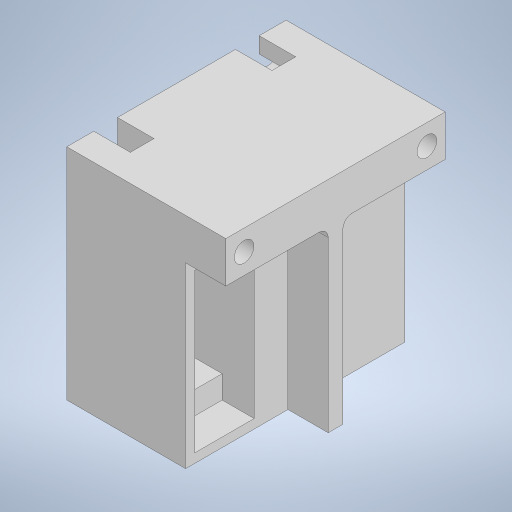
# Autodesk Inventor part: Part_2_servobox
Saved by Autodesk Inventor 2023 (Build 270158000, 158)
## iProperties
Created: 2023-09-29
Part Number: Part_2_servobox
Material: Generic
Document SubType Name: Modeling
Designer: zskus
Density: 1 g/cm^3
Appearance: Default
Author: zskus
Autodesk Inventor part; units mm, degrees
ref_plane "YZ Plane" through (0, 0, 0) normal (1, 0, 0) x (0, 1, 0)
ref_plane "XZ Plane" through (0, 0, 0) normal (0, 1, 0) x (-1, 0, 0)
ref_plane "XY Plane" through (0, 0, 0) normal (0, 0, 1) x (1, 0, 0)
sketch "Sketch1" plane through (0, 0, 0) normal (1, 0, 0) x (0, 1, 0)
  line L0 (38.1, 38.1) -> (-38.1, 38.1)
  line L1 (-38.1, 38.1) -> (-38.1, -38.1)
  line L2 (-38.1, -38.1) -> (38.1, -38.1)
  line L3 (38.1, -38.1) -> (38.1, 38.1)
  point P0 (0, 0)
  dimension "d0" = 76.2
  dimension "d1" = 76.2
  dimension "d2" = 38.1
  dimension "d3" = 38.1
  constraints: 8 end point, 2 parallel, 1 horizontal, 1 perpendicular
  measures "d0" distance of L2.end L0.start
  measures "d1" distance of L1.end L2.end
  measures "d2" distance from line of point (0, 0) L0
  measures "d3" distance from line of L3 point (0, 0)
extrude "Extrusion1" add sketch "Sketch1" along normal blind 41.275
sketch "Sketch2" plane through (41.275, 0, 0) normal (1, 0, 0) x (0, 0, -1)
  line L0 (-38.1, -38.1) -> (38.1, -38.1) projected
  line L1 (38.1, -38.1) -> (38.1, 38.1) projected
  line L2 (38.1, 38.1) -> (-38.1, 38.1) projected
  line L3 (-38.1, 38.1) -> (-38.1, -38.1) projected
  line L4 (-34.925, 17.4625) -> (-14.2875, 17.4625)
  line L5 (-14.2875, 17.4625) -> (-14.2875, -26.9875)
  line L6 (-14.2875, -26.9875) -> (-34.925, -26.9875)
  line L7 (-34.925, -26.9875) -> (-34.925, 17.4625)
  dimension "d64" = 20.6375
  dimension "d65" = 44.45
  dimension "d66" = 3.175
  dimension "d67" = 11.1125
  constraints: 8 end point, 2 parallel, 1 horizontal, 1 perpendicular
  measures "d64" distance of L4.start L4.end
  measures "d65" distance of L6.end L4.start
  measures "d66" distance between parallel lines of L3 L7
  measures "d67" distance between parallel lines of L0 L6
extrude "Extrusion2" cut sketch "Sketch2" against normal blind 39.6875 contours L4 L5 L6 L7
sketch "Sketch3" plane through (41.275, 0, 0) normal (1, 0, 0) x (0, 0, -1)
  line L0 (-14.2875, 17.4625) -> (-14.2875, -26.9875) projected
  line L1 (-14.2875, -26.9875) -> (-34.925, -26.9875) projected
  line L2 (-34.925, -26.9875) -> (-34.925, 17.4625) projected
  line L3 (-34.925, 17.4625) -> (-14.2875, 17.4625) projected
  line L4 (-38.1, -38.1) -> (38.1, -38.1) projected
  line L5 (38.1, -38.1) -> (38.1, 38.1) projected
  line L6 (38.1, 38.1) -> (-38.1, 38.1) projected
  line L7 (-38.1, 38.1) -> (-38.1, -38.1) projected
  line L8 (-14.2875, -26.9875) -> (-34.925, -26.9875) projected
  line L9 (-34.925, -26.9875) -> (-14.2875, -26.9875)
  line L10 (-14.2875, -26.9875) -> (-14.2875, -34.925)
  line L11 (-14.2875, -34.925) -> (-34.925, -34.925)
  line L12 (-34.925, -34.925) -> (-34.925, -26.9875)
  line L13 (-34.925, 17.4625) -> (-14.2875, 17.4625)
  line L14 (-14.2875, 17.4625) -> (-14.2875, 20.0025)
  line L15 (-14.2875, 20.0025) -> (-34.925, 20.0025)
  line L16 (-34.925, 20.0025) -> (-34.925, 17.4625)
  dimension "d68" = 7.9375
  dimension "d69" = 20.6375
  dimension "d70" = 20.6375
  dimension "d71" = 20.6375
  dimension "d72" = 2.54
  constraints: 16 end point, 4 parallel, 2 horizontal, 2 perpendicular
  measures "d68" distance of L9.end L10.end
  measures "d69" distance between parallel lines of L2 L0
  measures "d70" distance between parallel lines of L10 L12
  measures "d71" distance of L14.end L15.end
  measures "d72" distance between parallel lines of L3 L15
extrude "Extrusion3" cut sketch "Sketch3" against normal blind 11.1125 contours L3 L16 L15 L14 | L10 L11 L12 L1
sketch "Sketch4" plane through (15.875, 17.4625, 12.7) normal (0, -1, 0) x (1, 0, 0)
  line L0 (-15.875, -50.8) -> (-15.875, 25.4) projected
  line L1 (-15.875, 25.4) -> (25.4, 25.4) projected
  line L2 (25.4, -50.8) -> (25.4, 25.4) projected
  line L3 (-15.875, -50.8) -> (25.4, -50.8) projected
  line L4 (25.4, 22.225) -> (25.4, 1.5875) projected
  line L5 (25.4, 22.225) -> (14.2875, 22.225) projected
  line L6 (14.2875, 22.225) -> (14.2875, 1.5875) projected
  line L7 (25.4, 1.5875) -> (14.2875, 1.5875) projected
  line L8 (-15.875, 16.0338) -> (-3.175, 16.0338)
  line L9 (-3.175, 16.0338) -> (-3.175, 7.7788)
  line L10 (-3.175, 7.7788) -> (-15.875, 7.7788)
  line L11 (-15.875, 7.7788) -> (-15.875, 16.0338)
  point P0 (-3.175, 11.9063)
  dimension "d73" = 8.255
  dimension "d74" = 12.7
  dimension "d75" = 20.6375
  dimension "d76" = 10.3187
  constraints: 8 end point, 2 parallel, 1 horizontal, 1 midpoint, 1 perpendicular, 1 point on line
  measures "d73" distance of L8.end L9.end
  measures "d74" distance of L8.start L8.end
  measures "d75" distance of L5.end L6.end
  measures "d76" distance from line of L5 point (-3.175, 11.906)
extrude "Extrusion4" cut sketch "Sketch4" against normal blind 38.1 contours L0 L8 L9 L10
mirror "Mirror1" about plane through (0, 0, 0) normal (0, 0, 1) of "Extrusion4"
sketch "Sketch5" plane through (41.275, 0, 0) normal (1, 0, 0) x (0, 0, -1)
  line L0 (-38.1, -38.1) -> (38.1, -38.1) projected
  line L1 (38.1, -38.1) -> (38.1, 38.1) projected
  line L2 (38.1, 38.1) -> (-38.1, 38.1) projected
  line L3 (-38.1, 38.1) -> (-38.1, -38.1) projected
  line L4 (-38.1, -38.1) -> (38.1, -38.1) projected
  line L5 (-2.54, -38.1) -> (2.54, -38.1)
  line L6 (2.54, -38.1) -> (2.54, 20.6375)
  line L7 (2.54, 23.8125) -> (-2.54, 23.8125)
  line L8 (-2.54, 20.6375) -> (-2.54, -38.1)
  line L9 (-38.1, 38.1) -> (-38.1, -38.1) projected
  line L10 (38.1, 38.1) -> (-38.1, 38.1)
  line L11 (-38.1, 38.1) -> (-38.1, 23.8125)
  line L12 (-38.1, 23.8125) -> (-5.715, 23.8125)
  line L13 (38.1, 23.8125) -> (38.1, 38.1)
  line L14 (5.715, 23.8125) -> (38.1, 23.8125)
  line L15 (2.54, 23.8125) -> (2.54, 23.8125)
  arc A0 (-2.54, 20.6375) -> (-5.715, 23.8125) centre (-5.715, 20.6375) ccw
  arc A1 (5.715, 23.8125) -> (2.54, 20.6375) centre (5.715, 20.6375) ccw
  line L16 (-14.2875, 20.0025) -> (-14.2875, -34.925) projected
  line L17 (-34.925, -34.925) -> (-34.925, 20.0025) projected
  line L18 (-14.2875, -34.925) -> (-34.925, -34.925) projected
  line L19 (-34.925, 20.0025) -> (-14.2875, 20.0025) projected
  point P0 (0, 0)
  point P1 (38.1, 23.8125)
  point P2 (-2.54, -38.1)
  dimension "d36" = 5.08
  dimension "d39" = 2.54
  dimension "d40" = 3.175
  dimension "d44" = 61.9125
  constraints: 20 end point, 6 parallel, 6 point on line, 4 point on circle, 4 tangent, 3 perpendicular, 2 centre point, 2 horizontal, 1 equal radius
  measures "d36" distance between parallel lines of L6 L8
  measures "d39" distance from line of point (0, 0) L8
  measures "d40" radius of A0
  measures "d44" distance between parallel lines of L0 L12
extrude "Extrusion5" add sketch "Sketch5" along normal blind 13.97 contours L8 A0 L12 L3 L2 L1 L14 A1 L6 L0
sketch "Sketch6" plane through (0, -38.1, 38.1) normal (0, 0, 1) x (1, 0, 0)
  line L0 (-11.1125, 84.1375) -> (53.975, 84.1375)
  line L1 (53.975, 84.1375) -> (53.975, -9.525)
  line L2 (53.975, -9.525) -> (-11.1125, -9.525)
  line L3 (-11.1125, -9.525) -> (-11.1125, 84.1375)
  point P0 (0, 38.1)
  constraints: 8 end point, 2 parallel, 1 horizontal, 1 perpendicular
extrude "Extrusion6" [suppressed]
sketch "Sketch7" plane through (3.175, 22.225, -11.2395) normal (0, 0, -1) x (-1, 0, 0)
  line L0 (3.175, 15.875) -> (3.175, -60.325) projected
  line L1 (-28.575, 0) -> (-12.7, 0) projected
  line L2 (3.175, 15.875) -> (3.175, -60.325) projected
  line L3 (3.175, -60.325) -> (-38.1, -60.325) projected
  line L4 (-38.1, 1.5875) -> (-38.1, -60.325) projected
  line L5 (-38.1, 1.5875) -> (-52.07, 1.5875) projected
  line L6 (-52.07, 15.875) -> (-52.07, 1.5875) projected
  line L7 (3.175, 15.875) -> (-52.07, 15.875) projected
  line L8 (3.175, 15.875) -> (-6.35, 15.875)
  line L9 (-6.35, 15.875) -> (-6.35, 0)
  line L10 (-6.35, 0) -> (3.175, 0)
  line L11 (3.175, 0) -> (3.175, 15.875)
  line L12 (-6.35, -1.5875) -> (-6.35, 15.875) projected
  line L13 (-6.35, 0) -> (3.175, 12.7)
  point P0 (3.175, -22.225)
  point P1 (3.175, 15.875)
  point P2 (-6.35, 15.875)
  dimension "d49" = 9.525
  dimension "d50" = 3.175
  constraints: 10 end point, 2 parallel, 2 point on line, 1 horizontal, 1 perpendicular
  measures "d49" distance of L10.end L9.end
  measures "d50" distance of L0.start L13.end
extrude "Extrusion7" [suppressed]
mirror "Mirror2" [suppressed]
sketch "Sketch8" plane through (0, 38.1, 38.1) normal (0, 1, 0) x (1, 0, 0)
  line L0 (9.525, 46.1645) -> (0, 46.1645) projected
  line L1 (0, 36.6395) -> (9.525, 36.6395) projected
  line L2 (15.875, 47.625) -> (15.875, 60.579) projected
  arc A0 (0, 36.6395) -> (0, 46.1645) centre (-0.8069, 41.402) ccw
  line L3 (0, 46.1645) -> (0, 36.6395)
  point P0 (0, 38.1)
  point P1 (3.175, 49.3395)
  point P2 (3.175, 58.8645)
  dimension "d53" = 4.8304
  constraints: 2 end point, 2 point on circle, 1 centre point, 1 vertical, 3 other
  measures "d53" radius of A0
extrude "Extrusion8" [suppressed]
mirror "Mirror3" [suppressed]
sketch "Sketch11" plane through (55.245, 0, 0) normal (1, 0, 0) x (0, 0, -1)
  circle A0 centre (-31.75, 30.9563) radius 3.429
  circle A1 centre (31.75, 30.9563) radius 3.429
  line L0 (5.715, 23.8125) -> (38.1, 23.8125) projected
  line L1 (38.1, 23.8125) -> (38.1, 38.1) projected
  line L2 (38.1, 38.1) -> (-38.1, 38.1) projected
  line L3 (-38.1, 38.1) -> (-38.1, 23.8125) projected
  line L4 (-38.1, 23.8125) -> (-5.715, 23.8125) projected
  arc A2 (-2.54, 20.6375) -> (-5.715, 23.8125) centre (-5.715, 20.6375) ccw projected
  line L5 (-2.54, 20.6375) -> (-2.54, -38.1) projected
  line L6 (-2.54, -38.1) -> (2.54, -38.1) projected
  line L7 (2.54, -38.1) -> (2.54, 20.6375) projected
  arc A3 (5.715, 23.8125) -> (2.54, 20.6375) centre (5.715, 20.6375) ccw projected
  point P0 (0, 0)
  point P1 (0, 38.1)
  dimension "d77" = 63.5
  dimension "d78" = 76.2
  dimension "d79" = 31.75
  dimension "d80" = 14.2875
  dimension "d81" = 7.1437
  dimension "d82" = 7.1437
  dimension "d83" = 6.858
  dimension "d84" = 6.858
  constraints: 2 centre point, 1 midpoint
  measures "d77" distance of A0.centre A1.centre
  measures "d78" distance of L1.end L2.end
  measures "d79" horizontal distance of A1.centre point (0, 38.1)
  measures "d80" distance of L0.end L1.end
  measures "d81" distance from line of L2 A1.centre
  measures "d82" distance from line of L2 A0.centre
  measures "d83" diameter of A1
  measures "d84" diameter of A0
extrude "Extrusion10" cut sketch "Sketch11" against normal through all contours A0 | A1
equation "\"d2\" = 0.5 * d0"
equation "\"d3\" = 0.5 * d1"
equation "\"d70\" = d69"
equation "\"d71\" = d69"
equation "\"d76\" = 0.5 * d75"
equation "\"d39\" = 0.5 * d36"
equation "\"d44\" = d43"
equation "\"d79\" = 0.5 * d77"
equation "\"d81\" = 0.5 * d80"
equation "\"d82\" = d81"
equation "\"d43\" = 61.9125"
body "Solid1"
